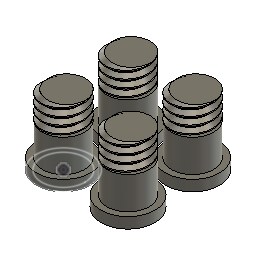
MyPad (Autodesk Fusion 360 archive; units mm, degrees)
design "Screws"
Autodesk Fusion 360 part; units mm, degrees
sketch "Sketch1" plane through (0, 0, 0) normal (0, 1, 0) x (1, 0, 0)
  circle A0 centre (0, 0) radius 2.5
  circle A1 centre (0, 0) radius 2
  dimension "d1" = 5
  dimension "d2" = 4
  constraint coincident A0.centre A1.centre
  measures "d1" diameter of A0
  measures "d2" diameter of A1
extrude "Extrude1" add sketch "Sketch1" along normal blind 1 contours A0 | A1 makes body 1
extrude "Extrude2" add sketch "Sketch1" along normal blind 6.5 contours A1 bodies 1
thread "Thread1" "ISO Metric profile 4.0 M4x0.7 M4x0.7 6g" major diameter 3.908 minor diameter 3.111 pitch 0.7 angle 60 modelled right hand crest width 0.1017 on face at (1.9901, 2.8333, -0.1991) from (0, 4, 0) to (0, 6.5, 0) crest through (1.954, 0.825, 0) on bodies 1
copy_body "CopyPasteBodies3" bodies 1 makes body 2
move_body "Move3" bodies 2 to x (1, 0, 0) y (0, 1, 0) z (0, 0, 1) at (6, 0, 0)
copy_body "CopyPasteBodies4" bodies 1 2 makes body 3 makes body 4
move_body "Move4" bodies 3 4 to x (1, 0, 0) y (0, 1, 0) z (0, 0, 1) at (0, 0, -6)
